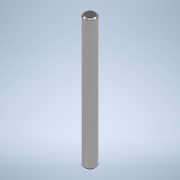
# Autodesk Inventor part: inox_89mm
Saved by Autodesk Inventor 2021 (Build 250183000, 183)
## iProperties
Created: 2021-04-05
Part Number: inox_89mm
Material: Generic
Document SubType Name: Modeling
Designer: jorge
Density: 1 g/cm^3
Appearance: Steel - Polished
Author: jorge
Autodesk Inventor part; units mm, degrees
ref_plane "YZ Plane" through (0, 0, 0) normal (1, 0, 0) x (0, 1, 0)
ref_plane "XZ Plane" through (0, 0, 0) normal (0, 1, 0) x (-1, 0, 0)
ref_plane "XY Plane" through (0, 0, 0) normal (0, 0, 1) x (1, 0, 0)
sketch "Sketch1" plane through (0, 0, 0) normal (0, 1, 0) x (-1, 0, 0)
  circle A0 centre (0, 0) radius 4
  dimension "d0" = 8
  constraints: 1 centre point, 1 coincident
  measures "d0" diameter of A0
extrude "Extrusion1" add sketch "Sketch1" along normal blind 89.5
chamfer "Chamfer1" distance 1 angle 45 2 edges at (4, 0, 0) (4, 89.5, 0)
body "Solid1"
